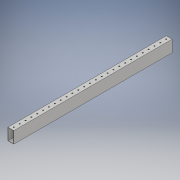
# Autodesk Inventor part: Front and Back Bar
Saved by Autodesk Inventor 2018 (Build 220112000, 112)
## iProperties
Created: 2020-05-06
Part Number: Front and Back Bar
Material: Generic
Document SubType Name: Modeling
Designer: maste
Density: 1 g/cm^3
Appearance: Default
Author: maste
Autodesk Inventor part; units mm, degrees
ref_plane "YZ Plane" through (0, 0, 0) normal (1, 0, 0) x (0, 1, 0)
ref_plane "XZ Plane" through (0, 0, 0) normal (0, 1, 0) x (-1, 0, 0)
ref_plane "XY Plane" through (0, 0, 0) normal (0, 0, 1) x (1, 0, 0)
sketch "Sketch1" plane through (0, 0, 0) normal (0, 0, 1) x (1, 0, 0)
  line L0 (0, 0) -> (25.4, 0)
  line L1 (25.4, 0) -> (25.4, 50.8)
  line L2 (25.4, 50.8) -> (0, 50.8)
  line L3 (0, 50.8) -> (0, 0)
  line L4 (1.5875, 49.2125) -> (23.8125, 49.2125)
  line L5 (23.8125, 49.2125) -> (23.8125, 1.5875)
  line L6 (23.8125, 1.5875) -> (1.5875, 1.5875)
  line L7 (1.5875, 1.5875) -> (1.5875, 49.2125)
  dimension "d0" = 25.4
  dimension "d1" = 50.8
  dimension "d2" = 1.5875
  constraints: 16 end point, 4 parallel, 2 perpendicular, 1 horizontal, 3 other
  measures "d0" distance of L2.end L1.end
  measures "d1" distance of L1.end L0.end
  measures "d2" distance between parallel lines of L2 L4
extrude "Extrusion1" add sketch "Sketch1" along normal blind 685.8
sketch "Sketch2" plane through (0, 50.8, 0) normal (0, 1, 0) x (1, 0, 0)
  line L0 (23.8125, 0) -> (1.5875, 0) construction
  line L1 (12.7, 0) -> (12.7, -12.7) construction
  line L2 (12.7, -12.7) -> (12.7, -38.1) construction
  line L3 (12.7, -38.1) -> (12.7, -63.5) construction
  line L4 (12.7, -63.5) -> (12.7, -88.9) construction
  line L5 (12.7, -88.9) -> (12.7, -114.3) construction
  line L6 (12.7, -114.3) -> (12.7, -139.7) construction
  line L7 (12.7, -139.7) -> (12.7, -165.1) construction
  line L8 (12.7, -165.1) -> (12.7, -190.5) construction
  line L9 (12.7, -190.5) -> (12.7, -215.9) construction
  line L10 (12.7, -215.9) -> (12.7, -241.3) construction
  line L11 (12.7, -241.3) -> (12.7, -266.7) construction
  line L12 (12.7, -266.7) -> (12.7, -292.1) construction
  line L13 (12.7, -292.1) -> (12.7, -317.5) construction
  line L14 (12.7, -317.5) -> (12.7, -342.9) construction
  line L15 (12.7, -342.9) -> (12.7, -368.3) construction
  line L16 (12.7, -368.3) -> (12.7, -393.7) construction
  line L17 (12.7, -393.7) -> (12.7, -419.1) construction
  line L18 (12.7, -419.1) -> (12.7, -444.5) construction
  line L19 (12.7, -444.5) -> (12.7, -469.9) construction
  line L20 (12.7, -469.9) -> (12.7, -495.3) construction
  line L21 (12.7, -495.3) -> (12.7, -469.9) construction
  line L22 (12.7, -469.9) -> (12.7, -495.3) construction
  line L23 (12.7, -495.3) -> (12.7, -520.7) construction
  line L24 (12.7, -520.7) -> (12.7, -546.1) construction
  line L25 (12.7, -546.1) -> (12.7, -571.5) construction
  line L26 (12.7, -571.5) -> (12.7, -596.9) construction
  line L27 (12.7, -596.9) -> (12.7, -622.3) construction
  line L28 (12.7, -622.3) -> (12.7, -647.7) construction
  line L29 (12.7, -647.7) -> (12.7, -673.1) construction
  circle A0 centre (12.7, -673.1) radius 2.5781
  circle A1 centre (12.7, -647.7) radius 2.5781
  circle A2 centre (12.7, -622.3) radius 2.5781
  circle A3 centre (12.7, -596.9) radius 2.5781
  circle A4 centre (12.7, -571.5) radius 2.5781
  circle A5 centre (12.7, -546.1) radius 2.5781
  circle A6 centre (12.7, -520.7) radius 2.5781
  circle A7 centre (12.7, -495.3) radius 2.5781
  circle A8 centre (12.7, -469.9) radius 2.5781
  circle A9 centre (12.7, -444.5) radius 2.5781
  circle A10 centre (12.7, -419.1) radius 2.5781
  circle A11 centre (12.7, -393.7) radius 2.5781
  circle A12 centre (12.7, -368.3) radius 2.5781
  circle A13 centre (12.7, -342.9) radius 2.5781
  circle A14 centre (12.7, -317.5) radius 2.5781
  circle A15 centre (12.7, -292.1) radius 2.5781
  circle A16 centre (12.7, -266.7) radius 2.5781
  circle A17 centre (12.7, -241.3) radius 2.5781
  circle A18 centre (12.7, -215.9) radius 2.5781
  circle A19 centre (12.7, -190.5) radius 2.5781
  circle A20 centre (12.7, -165.1) radius 2.5781
  circle A21 centre (12.7, -139.7) radius 2.5781
  circle A22 centre (12.7, -114.3) radius 2.5781
  circle A23 centre (12.7, -88.9) radius 2.5781
  circle A24 centre (12.7, -63.5) radius 2.5781
  circle A25 centre (12.7, -38.1) radius 2.5781
  circle A26 centre (12.7, -12.7) radius 2.5781
  point P0 (0, 0)
  dimension "d5" = 12.7
  dimension "d6" = 25.4
  dimension "d7" = 25.4
  dimension "d8" = 25.4
  dimension "d9" = 25.4
  dimension "d10" = 25.4
  dimension "d11" = 25.4
  dimension "d12" = 25.4
  dimension "d13" = 25.4
  dimension "d14" = 25.4
  dimension "d15" = 25.4
  dimension "d16" = 25.4
  dimension "d17" = 25.4
  dimension "d18" = 25.4
  dimension "d19" = 25.4
  dimension "d20" = 25.4
  dimension "d21" = 25.4
  dimension "d22" = 25.4
  dimension "d23" = 25.4
  dimension "d24" = 25.4
  dimension "d25" = 25.4
  dimension "d26" = 25.4
  dimension "d27" = 25.4
  dimension "d28" = 25.4
  dimension "d29" = 25.4
  dimension "d30" = 25.4
  dimension "d31" = 25.4
  dimension "d32" = 25.4
  dimension "d33" = 25.4
  dimension "d34" = 5.1562
  dimension "d35" = 5.1562
  dimension "d36" = 5.1562
  dimension "d37" = 5.1562
  dimension "d38" = 5.1562
  dimension "d39" = 5.1562
  dimension "d40" = 5.1562
  dimension "d41" = 5.1562
  dimension "d42" = 5.1562
  dimension "d43" = 5.1562
  dimension "d44" = 5.1562
  dimension "d45" = 5.1562
  dimension "d46" = 5.1562
  dimension "d47" = 5.1562
  dimension "d48" = 5.1562
  dimension "d49" = 5.1562
  dimension "d50" = 5.1562
  dimension "d51" = 5.1562
  dimension "d52" = 5.1562
  dimension "d53" = 5.1562
  dimension "d54" = 5.1562
  dimension "d55" = 5.1562
  dimension "d56" = 5.1562
  dimension "d57" = 5.1562
  dimension "d58" = 5.1562
  dimension "d59" = 5.1562
  dimension "d60" = 5.1562
  constraints: 58 end point, 27 centre point, 26 point on line, 2 collinear, 1 coincident, 1 midpoint, 1 vertical
  measures "d5" distance of L1.start L1.end
  measures "d6" distance of L1.end L2.end
  measures "d7" distance of L2.end L3.end
  measures "d8" distance of L3.end L4.end
  measures "d9" distance of L4.end L5.end
  measures "d10" distance of L5.end L6.end
  measures "d11" distance of L6.end L7.end
  measures "d12" distance of L7.end L8.end
  measures "d13" distance of L8.end L9.end
  measures "d14" distance of L9.end L10.end
  measures "d15" distance of L10.end L11.end
  measures "d16" distance of L11.end L12.end
  measures "d17" distance of L12.end L13.end
  measures "d18" distance of L13.end L14.end
  measures "d19" distance of L14.end L15.end
  measures "d20" distance of L15.end L16.end
  measures "d21" distance of L16.end L17.end
  measures "d22" distance of L17.end L18.end
  measures "d23" distance of L18.end L19.end
  measures "d24" distance of L19.end L20.end
  measures "d25" distance of L20.end L19.end
  measures "d26" distance of L19.end L20.end
  measures "d27" distance of L20.end L23.end
  measures "d28" distance of L23.end L24.end
  measures "d29" distance of L24.end L25.end
  measures "d30" distance of L25.end L26.end
  measures "d31" distance of L26.end L27.end
  measures "d32" distance of L27.end L28.end
  measures "d33" distance of L28.end L29.end
  measures "d34" diameter of A0
  measures "d35" diameter of A1
  measures "d36" diameter of A2
  measures "d37" diameter of A3
  measures "d38" diameter of A4
  measures "d39" diameter of A5
  measures "d40" diameter of A6
  measures "d41" diameter of A7
  measures "d42" diameter of A8
  measures "d43" diameter of A9
  measures "d44" diameter of A10
  measures "d45" diameter of A11
  measures "d46" diameter of A12
  measures "d47" diameter of A13
  measures "d48" diameter of A14
  measures "d49" diameter of A15
  measures "d50" diameter of A16
  measures "d51" diameter of A17
  measures "d52" diameter of A18
  measures "d53" diameter of A19
  measures "d54" diameter of A20
  measures "d55" diameter of A21
  measures "d56" diameter of A22
  measures "d57" diameter of A23
  measures "d58" diameter of A24
  measures "d59" diameter of A25
  measures "d60" diameter of A26
extrude "Extrusion2" cut sketch "Sketch2" against normal blind 685.8
body "Solid1"
